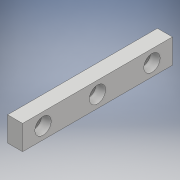
# Autodesk Inventor part: rail_SSEB10
Saved by Autodesk Inventor 2018.3 (Build 223284000, 284)
## iProperties
Created: 2018-05-24
Part Number: rail_SSEB10
Material: 一般
Document SubType Name: Modeling
Designer: Shin
Density: 1 g/cm^3
Appearance: 既定
Author: Shin
Autodesk Inventor part; units mm, degrees
ref_plane "YZ Plane" through (0, 0, 0) normal (1, 0, 0) x (0, 1, 0)
ref_plane "XZ Plane" through (0, 0, 0) normal (0, 1, 0) x (-1, 0, 0)
ref_plane "XY Plane" through (0, 0, 0) normal (0, 0, 1) x (1, 0, 0)
sketch "スケッチ1" plane through (0, 0, 0) normal (0, 1, 0) x (-1, 0, 0)
  line L0 (0, 0) -> (5.5, 0)
  line L1 (5.5, 0) -> (5.5, -9)
  line L2 (5.5, -9) -> (0, -9)
  line L3 (0, -9) -> (0, 0)
  dimension "d0" = 5.5
  dimension "d1" = 9
  constraints: 8 end point, 2 parallel, 1 horizontal, 1 perpendicular
  measures "d0" distance of L1.end L2.end
  measures "d1" distance of L0.end L1.end
extrude "押し出し1" add sketch "スケッチ1" along normal blind 55
sketch "スケッチ2" plane through (0, 0, 0) normal (1, 0, 0) x (0, 0, -1)
  line L0 (0, 55) -> (9, 55) projected
  line L1 (4.5, 55) -> (4.5, 0)
  line L2 (9, 0) -> (0, 0) projected
  point P0 (4.5, 27.5)
  point P1 (4.5, 47.5)
  point P2 (4.5, 7.5)
  dimension "d4" = 27.5
  dimension "d5" = 20
  dimension "d6" = 20
  constraints: 3 midpoint, 2 end point, 2 point on line
  measures "d4" distance from line of point (4.5, 27.5) L0
  measures "d5" distance of point (4.5, 27.5) point (4.5, 47.5)
  measures "d6" distance of point (4.5, 27.5) point (4.5, 7.5)
hole "穴1" at (0, 27.5, -4.5) at (0, 47.5, -4.5) at (0, 7.5, -4.5) direction (-1, 0, 0) diameter 3.5 depth 8 tip angle 118 counterbore diameter 6 counterbore depth 3.5
